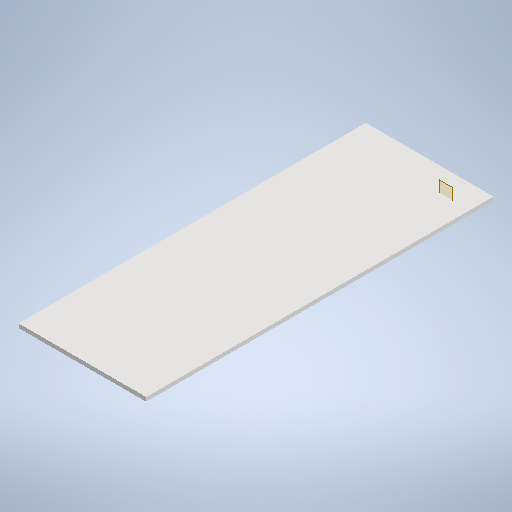
# Autodesk Inventor part: Payload Plate
Saved by Autodesk Inventor 2025 (Build 290162000, 162)
## iProperties
Created: 2024-09-16
Part Number: Payload Plate
Material: Generic
Document SubType Name: Modeling
Designer: Cupri
Density: 1 g/cm^3
Appearance: Default
Mass: 7091.63 g
Surface Area: 3606.68 cm^2
Volume: 7091.63 cm^3
Author: Cupri
Autodesk Inventor part; units mm, degrees
ref_plane "YZ Plane" through (0, 0, 0) normal (1, 0, 0) x (0, 1, 0)
ref_plane "Work Plane2" through (-165.1, -76.2, 552.7548) normal (0, 0, -1) x (0, 1, 0)
ref_plane "Work Plane3" through (0, 0, 37.3534) normal (0, 0, 1) x (1, 0, 0)
sketch "Sketch1" plane through (0, 0, 37.3534) normal (0, 0, 1) x (1, 0, 0)
  line L0 (-114.3, -6.2716) -> (-12.7, -6.2716) projected
  line L1 (-127, -49.1085) -> (-127, -74.5085) projected
  arc A0 (-127, -74.5085) -> (-114.3, -76.1216) centre (-114.3, -25.3216) ccw projected
  line L2 (-12.7, -76.1216) -> (-114.3, -76.1216) projected
  arc A1 (-12.7, -76.1216) -> (0, -74.5085) centre (-12.7, -25.3216) ccw projected
  line L3 (0, -74.5085) -> (0, -49.1085) projected
  line L4 (0, -49.1085) -> (12.7, -49.1085) projected
  line L5 (12.7, -49.1085) -> (12.7, -69.3157) projected
  arc A2 (12.7, -69.3157) -> (38.1, -25.3216) centre (-12.7, -25.3216) ccw projected
  line L6 (38.1, 0.0784) -> (38.1, -25.3216) projected
  arc A3 (38.1, 0.0784) -> (-38.1, 76.2784) centre (-38.1, 0.0784) ccw projected
  line L7 (-38.1, 76.2784) -> (-12.7, -6.2716) projected
  line L8 (-12.7, -6.2716) -> (-114.3, -6.2716) projected
  line L9 (-114.3, -6.2716) -> (-88.9, 76.2784) projected
  arc A4 (-88.9, 76.2784) -> (-165.1, 0.0784) centre (-88.9, 0.0784) ccw projected
  line L10 (-165.1, -25.3216) -> (-165.1, 0.0784) projected
  arc A5 (-165.1, -25.3216) -> (-139.7, -69.3157) centre (-114.3, -25.3216) ccw projected
  line L11 (-139.7, -69.3157) -> (-139.7, -49.1085) projected
  line L12 (-139.7, -49.1085) -> (-127, -49.1085) projected
  line L13 (38.1, 0.0784) -> (38.1, -25.3216) projected
  line L14 (-63.5, -6.2716) -> (38.1, -6.2716)
  line L15 (-123.5, -12.6216) -> (0, -12.6216) projected
  line L16 (-63.5, -12.6216) -> (38.1, -12.6216)
  line L17 (38.1, -12.6216) -> (38.1, -6.2716)
  line L18 (-63.5, -6.2716) -> (-63.5, -12.6216) construction
  line L19 (-12.7, -6.2716) -> (-114.3, -6.2716)
  line L20 (-63.5, -6.2716) -> (-165.1, -6.2716)
  line L21 (-63.5, -12.6216) -> (-165.1, -12.6216)
  line L22 (-165.1, -12.6216) -> (-165.1, -6.2716)
  point P0 (0, 0)
  point P1 (-165.1, -12.6216)
  point P2 (-123.5, -12.7)
  point P3 (38.1, -6.2716)
  point P4 (-165.1, -6.2716)
  constraints: 16 end point, 4 symmetric about line, 2 midpoint, 2 point on line, 1 collinear, 1 parallel, 1 perpendicular
extrude "Extrusion1" add sketch "Sketch1" along normal up to surface (515.4014 mm away) contours L0 L14 L6 L16 L15 L21 L10 L20
sketch "Sketch2" plane through (0, 0, 37.3534) normal (0, 0, -1) x (-1, 0, 0)
  line L0 (165.1, -12.6216) -> (-38.1, -12.6216) projected
  line L1 (165.1, -6.2716) -> (165.1, -12.6216) projected
  line L2 (-38.1, -6.2716) -> (165.1, -6.2716) projected
  line L3 (-38.1, -12.6216) -> (-38.1, -6.2716) projected
  point P0 (0, 0)
ref_plane "Work Plane4" through (-165.1, -76.1216, 0) normal (0, 0, 1) x (1, 0, 0)
extrude "Extrusion2" add sketch "Sketch2" along normal up to surface (37.3534 mm away)
body "Solid1"
